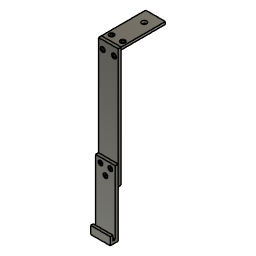
DirectionEncoderBarSupport_PESTA (Autodesk Fusion 360 design; units mm, degrees)
Autodesk Fusion 360 part; units mm, degrees
sketch "Sketch1" plane through (0, 0, 0) normal (0, 0, 1) x (1, 0, 0) in component "GanchoInferior"
  line L0 (20, 8) -> (-20, 8)
  line L1 (-20, 8) -> (-20, -8)
  line L2 (-20, -8) -> (20, -8)
  line L3 (20, -8) -> (20, 8)
  line L4 (20, 8) -> (-20, -8) construction
  line L5 (-20, 8) -> (20, -8) construction
  dimension "d1" = 40
  dimension "d2" = 16
  constraint horizontal L0
  constraint perpendicular L0 L1
  constraint parallel L0 L2
  constraint parallel L1 L3
  constraint coincident L4 origin
  constraint coincident L5 origin
  measures "d1" distance of L1.end L2.end
  measures "d2" distance of L0.end L1.end
extrude "Extrude1" add sketch "Sketch1" along normal blind 6 makes body 1 in component "GanchoInferior"
sketch "Sketch2" plane through (0, 0, 6) normal (0, 0, 1) x (-1, 0, 0) in component "GanchoInferior"
  line L0 (-20, 8) -> (-20, -8)
  line L1 (-20, -8) -> (20, -8)
  line L2 (20, -8) -> (20, 8)
  line L3 (20, 8) -> (-20, 8)
  line L4 (20, -8) -> (-20, -8)
  line L5 (-20, -8) -> (-20, -2)
  line L6 (-20, -2) -> (20, -2)
  line L7 (20, -2) -> (20, -8)
  line L8 (20, 8) -> (-20, 8)
  line L9 (-20, 8) -> (-20, 2.7)
  line L10 (-20, 2.7) -> (20, 2.7)
  line L11 (20, 2.7) -> (20, 8)
  dimension "d5" = 6
  dimension "d6" = 4.7
  constraint horizontal L4
  constraint vertical L5
  constraint horizontal L6
  constraint vertical L7
  constraint coincident L0 L5.end
  constraint coincident L1.end L2.start
  constraint horizontal L8
  constraint vertical L9
  constraint horizontal L10
  constraint vertical L11
  constraint coincident L0 L9.end
  constraint coincident L2.end L3.start
  measures "d5" distance of L1.end L6.end
  measures "d6" distance of L6 L10
extrude "Extrude2" add sketch "Sketch2" along normal blind 130 contours L0 L1 L2 L4 L5 L6 L7 bodies 1 in component "GanchoInferior"
extrude "Extrude3" add sketch "Sketch2" along normal blind 10 contours L0 L2 L3 L8 L9 L10 L11 bodies 1 in component "GanchoInferior"
sketch "Sketch3" plane through (0, 8, 0) normal (0, -1, 0) x (1, 0, 0) in component "GanchoInferior"
  line L0 (-20, 6) -> (20, 6)
  line L1 (20, 6) -> (20, 136)
  line L2 (20, 136) -> (-20, 136)
  line L3 (-20, 136) -> (-20, 6)
  circle A0 centre (10, 126) radius 4.75
  circle A1 centre (-10, 126) radius 4.75
  circle A2 centre (-10, 126) radius 1.8
  circle A3 centre (10, 126) radius 1.8
  line L4 (10, 126) -> (-10, 126)
  line L5 (10, 126) -> (0, 108.6795)
  line L6 (0, 108.6795) -> (-10, 126)
  circle A4 centre (0, 108.6795) radius 1.8
  circle A5 centre (0, 108.6795) radius 4.75
  line L7 (20, 0) -> (-20, 0)
  line L8 (-20, 0) -> (-20, 136)
  line L9 (-20, 136) -> (20, 136)
  line L10 (20, 136) -> (20, 0)
  point P0 (0, 126)
  dimension "d12" = 9.5
  dimension "d13" = 3.6
  dimension "d14" = 120
  dimension "d15" = 20
  constraint concentric A1 A2
  constraint concentric A0 A3
  constraint equal A2 A3
  constraint equal A0 A1
  constraint coincident A0.centre A3.centre
  constraint coincident A1.centre A2.centre
  constraint horizontal L4
  constraint midpoint L4 P0
  constraint vertical origin P0
  constraint equal L4 L6
  constraint equal L5 L6
  constraint coincident L5.end L6.start
  constraint concentric A4 A5
  constraint equal A0 A5
  constraint equal A3 A4
  measures "d12" diameter of A1
  measures "d13" diameter of A2
  measures "d14" distance of L0 A0.centre
  measures "d15" distance of A0.centre A1.centre
extrude "Extrude4" cut sketch "Sketch3" along normal blind 6 contours A3 L4 L5 | A3 L4 L5 | A2 L4 L6 | A2 L4 L6 | L5 L6 A4 | L5 L6 A4 bodies 1 in component "GanchoInferior"
extrude "Extrude5" cut sketch "Sketch3" against normal blind 2 from surface at 6 contours A0 A3 L4 L5 | A0 A3 L4 L5 | A1 A2 L4 L6 | A1 A2 L4 L6 | L5 L6 A4 A5 | L5 L6 A4 A5 bodies 1 in component "GanchoInferior"
sketch "Sketch1 (2)" plane through (0, 2, 0) normal (0, -1, 0) x (1, 0, 0) in component "Coluna"
  line L0 (-20, 6) -> (20, 6)
  line L1 (20, 6) -> (20, 136)
  line L2 (20, 136) -> (-20, 136)
  line L3 (-20, 136) -> (-20, 6)
  line L4 (-20, 96) -> (20, 96)
  line L5 (20, 96) -> (20, 339)
  line L6 (20, 339) -> (-20, 339)
  line L7 (-20, 339) -> (-20, 96)
  circle A0 centre (-10, 126) radius 4.75
  circle A1 centre (0, 108.6795) radius 4.75
  circle A2 centre (10, 126) radius 4.75
  dimension "d20" = 40
  constraint horizontal L4
  constraint vertical L5
  constraint horizontal L6
  constraint vertical L7
  constraint coincident L3 L4.start
  constraint coincident L1 L4.end
  measures "d20" distance of L2 L4
extrude "Extrude1'" add sketch "Sketch1 (2)" along normal blind 6 separate body contours L1 L2 L3 L4 L5 L7 | L2 L5 L6 L7 | A0 | A1 | A2 makes body 2 in component "Coluna"
extrude "Extrude2'" cut sketch "Sketch3" along normal blind 12 contours A3 L4 L5 | A3 L4 L5 | A2 L4 L6 | A2 L4 L6 | L5 L6 A4 | L5 L6 A4 bodies 2 in component "Coluna"
sketch "Sketch2 (2)" plane through (0, -4, 0) normal (0, -1, 0) x (1, 0, 0) in component "Coluna"
  line L0 (-20, 339) -> (-20, 96)
  line L1 (-20, 96) -> (20, 96)
  line L2 (20, 96) -> (20, 339)
  line L3 (20, 339) -> (-20, 339)
  circle A0 centre (10, 126) radius 4.75
  circle A1 centre (-10, 126) radius 4.75
  circle A2 centre (0, 108.6795) radius 4.75
  circle A3 centre (10, 126) radius 1.8
  circle A4 centre (0, 108.6795) radius 1.8
  circle A5 centre (-10, 126) radius 1.8
  dimension "d26" = 9.5
  constraint equal A0 A1
  constraint equal A1 A2
  measures "d26" diameter of A0
extrude "Extrude3'" cut sketch "Sketch2 (2)" against normal blind 2 contours A0 | A1 | A2 | A3 | A4 | A5 bodies 2 in component "Coluna"
sketch "Sketch3 (2)" plane through (0, -4, 0) normal (0, -1, 0) x (1, 0, 0) in component "Coluna"
  circle A0 centre (-10, 126) radius 4.75
  circle A1 centre (0, 108.6795) radius 4.75
  circle A2 centre (10, 126) radius 4.75
  line L0 (-20, 339) -> (-20, 96)
  line L1 (-20, 96) -> (20, 96)
  line L2 (20, 96) -> (20, 339)
  line L3 (20, 339) -> (-20, 339)
  line L4 (-20, 332) -> (-3, 332)
  line L5 (-3, 332) -> (-3, 312)
  line L6 (-3, 312) -> (-20, 312)
  line L7 (-20, 312) -> (-20, 332)
  line L8 (20, 332) -> (3, 332)
  line L9 (3, 332) -> (3, 312)
  line L10 (3, 312) -> (20, 312)
  line L11 (20, 312) -> (20, 332)
  circle A3 centre (-11.5, 322) radius 2.5
  circle A4 centre (11.5, 322) radius 2.5
  point P0 (-11.5, 332)
  point P1 (-20, 322)
  point P2 (3, 322)
  point P3 (11.5, 332)
  dimension "d29" = 17
  dimension "d30" = 20
  dimension "d31" = 7
  dimension "d32" = 5
  dimension "d33" = 5
  constraint horizontal L4
  constraint vertical L5
  constraint horizontal L6
  constraint vertical L7
  constraint coincident L0 L4.start
  constraint horizontal L8
  constraint vertical L9
  constraint horizontal L10
  constraint vertical L11
  constraint coincident L2 L8.start
  constraint equal L4 L8
  constraint equal L5 L9
  constraint horizontal L4.end L8.end
  constraint midpoint L4 P0
  constraint midpoint L7 P1
  constraint midpoint L9 P2
  constraint midpoint L8 P3
  constraint vertical A3.centre P0
  constraint horizontal A3.centre P1
  constraint horizontal A4.centre P2
  constraint vertical A4.centre P3
  measures "d29" distance of L4.start L4.end
  measures "d30" distance of L4.start L6.end
  measures "d31" distance of L3 L4
  measures "d32" diameter of A3
  measures "d33" diameter of A4
extrude "Extrude4'" cut sketch "Sketch3 (2)" against normal blind 6 contours A3 | A4 bodies 2 in component "Coluna"
sketch "Sketch4" plane through (0, 2, 0) normal (0, 1, 0) x (-1, 0, 0) in component "Coluna"
  circle A0 centre (11.5, 322) radius 2.5
  circle A1 centre (-11.5, 322) radius 2.5
  circle A2 centre (-10, 126) radius 1.8
  circle A3 centre (0, 108.6795) radius 1.8
  circle A4 centre (10, 126) radius 1.8
  line L0 (20, 96) -> (20, 339)
  line L1 (20, 339) -> (-20, 339)
  line L2 (-20, 339) -> (-20, 96)
  line L3 (-20, 96) -> (20, 96)
  circle A5 centre (-11.5, 322) radius 4.75
  circle A6 centre (11.5, 322) radius 4.75
  dimension "d36" = 9.5
  dimension "d37" = 9.5
  constraint concentric A1 A5
  constraint concentric A0 A6
  measures "d36" diameter of A5
  measures "d37" diameter of A6
extrude "Extrude5'" cut sketch "Sketch4" against normal blind 0.5 contours A5 | A6 bodies 2 in component "Coluna"
sketch "Sketch1 (3)" plane through (0, -4, 0) normal (0, -1, 0) x (1, 0, 0) in component "Ponte"
  circle A0 centre (-11.5, 322) radius 2.5
  circle A1 centre (11.5, 322) radius 2.5
  circle A2 centre (-10, 126) radius 4.75
  circle A3 centre (0, 108.6795) radius 4.75
  circle A4 centre (10, 126) radius 4.75
  line L0 (-20, 339) -> (-20, 96)
  line L1 (-20, 96) -> (20, 96)
  line L2 (20, 96) -> (20, 339)
  line L3 (20, 339) -> (-20, 339)
  line L4 (-20, 339) -> (20, 339)
  line L5 (20, 339) -> (20, 334)
  line L6 (20, 334) -> (-20, 334)
  line L7 (-20, 334) -> (-20, 339)
  dimension "d40" = 5
  constraint horizontal L4
  constraint vertical L5
  constraint horizontal L6
  constraint vertical L7
  constraint coincident L0.start L3.end
  measures "d40" distance of L0.start L6.end
extrude "Extrude1''" add sketch "Sketch1 (3)" along normal blind 90 separate body contours L0 L2 L3 L4 L5 L6 L7 makes body 3 in component "Ponte"
sketch "Sketch2 (3)" plane through (0, 0, 339) normal (0, 0, 1) x (-1, 0, 0) in component "Ponte"
  line L0 (-20, 4) -> (20, 4)
  line L1 (20, 4) -> (20, 94)
  line L2 (20, 94) -> (-20, 94)
  line L3 (-20, 94) -> (-20, 4)
  line L4 (20, 4) -> (3, 4)
  line L5 (3, 4) -> (3, 24)
  line L6 (3, 24) -> (20, 24)
  line L7 (20, 24) -> (20, 4)
  circle A0 centre (11.5, 16) radius 2.5
  circle A1 centre (-11.5, 16) radius 2.5
  circle A2 centre (11.5, 16) radius 4.75
  circle A3 centre (-11.5, 16) radius 4.75
  line L8 (-20, 26) -> (-3, 26)
  line L9 (-3, 26) -> (-3, 6)
  line L10 (-3, 6) -> (-20, 6)
  line L11 (-20, 6) -> (-20, 26)
  point P0 (11.5, 4)
  point P1 (-11.5, 6)
  point P2 (-3, 16)
  dimension "d43" = 17
  dimension "d44" = 20
  dimension "d47" = 5
  dimension "d48" = 5
  dimension "d51" = 9.5
  dimension "d52" = 9.5
  dimension "d72" = 17
  dimension "d73" = 20
  dimension "d74" = 2
  constraint horizontal L4
  constraint vertical L5
  constraint horizontal L6
  constraint vertical L7
  constraint coincident L0.end L1.start
  constraint midpoint L4 P0
  constraint horizontal A0.centre P2
  constraint horizontal A1.centre P2
  constraint vertical A1.centre P1
  constraint vertical A0.centre P0
  constraint concentric A0 A2
  constraint concentric A1 A3
  constraint horizontal L8
  constraint vertical L9
  constraint horizontal L10
  constraint vertical L11
  constraint coincident L3 L8.start
  constraint midpoint P2 L9
  constraint coincident P1 L10
  constraint midpoint P1 L10
  measures "d43" distance of L0.end L4.end
  measures "d44" distance of L0.end L6.end
  measures "d47" diameter of A0
  measures "d48" diameter of A1
  measures "d51" diameter of A2
  measures "d52" diameter of A3
  measures "d72" distance of L8.start L8.end
  measures "d73" distance of L8.start L10.end
  measures "d74" distance of L0 L10
extrude "Extrude2''" cut sketch "Sketch2 (3)" against normal blind 5 contours A0 | A1 bodies 3 in component "Ponte"
extrude "Extrude3''" cut sketch "Sketch2 (3)" against normal blind 0.5 contours A2 | A3 bodies 3 in component "Ponte"
sketch "Sketch3 (3)" plane through (0, 0, 339) normal (0, 0, 1) x (-1, 0, 0) in component "Ponte"
  circle A0 centre (11.5, 16) radius 4.75
  circle A1 centre (-11.5, 16) radius 4.75
  line L0 (-20, 4) -> (20, 4)
  line L1 (20, 4) -> (20, 94)
  line L2 (20, 94) -> (-20, 94)
  line L3 (-20, 94) -> (-20, 4)
  circle A2 centre (0, 71) radius 5
  dimension "d55" = 67
  dimension "d56" = 10
  constraint vertical origin A2.centre
  measures "d55" distance of L0 A2.centre
  measures "d56" diameter of A2
extrude "Extrude4''" cut sketch "Sketch3 (3)" against normal blind 5 contours A2 bodies 3 in component "Ponte"
move_body "Move1" bodies 2 to x (-1, 0, 0) y (0, -1, 0) z (0, 0, 1) at (-0.2927, 4, 0) in component "Coluna"
move_body "Move1'" bodies 3 to x (-1, 0, 0) y (0, -1, 0) z (0, 0, 1) at (0, -98, 0) in component "Ponte"
component "GanchoInferior" placed x (1, 0, 0) y (0, 1, 0) z (0, 0, 1) at (0, 0, 0)
component "Coluna" placed x (1, 0, 0) y (0, 1, 0) z (0, 0, 1) at (0.2927, 6, 0)
component "Ponte" placed x (1, 0, 0) y (0, 1, 0) z (0, 0, 1) at (0, 108, 0)
